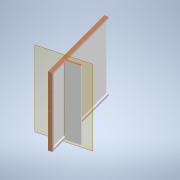
# Autodesk Inventor part: ДИ 00.00.09
Saved by Autodesk Inventor 2021.2 (Build 252289000, 289)
## iProperties
Created: 2021-10-12
Part Number: ДИ 00.00.09
Material: Типовые
Document SubType Name: Modeling
Designer: Surflay
Density: 1 g/cm^3
Appearance: По умолчанию
Author: Surflay
Autodesk Inventor part; units mm, degrees
ref_plane "YZ Plane" through (0, 0, 0) normal (1, 0, 0) x (0, 1, 0)
ref_plane "XZ Plane" through (0, 0, 0) normal (0, 1, 0) x (-1, 0, 0)
ref_plane "XY Plane" through (0, 0, 0) normal (0, 0, 1) x (1, 0, 0)
ref_plane "РабПлоскость1" through (-45, 39.0097, 0) normal (-0.9659258, 0, 0.258819) x (0, -1, 0)
sketch "Эскиз1" plane through (-45, 39.0097, 0) normal (-0.9659258, 0, 0.258819) x (0, -1, 0)
  line L0 (0, 0) -> (78.0194, 0) projected
  line L1 (0.0194, 85.4597) -> (78.0194, 85.4597) projected
  line L2 (78.0194, 68.8953) -> (78.0194, 85.4597) projected
  line L3 (-2.9723, 68.8953) -> (78.0194, 68.8953) projected
  line L4 (-2.9723, 68.8953) -> (-2.9723, 74.9718) projected
  ellipse E0 centre (-19.9806, 77.6951) end of major axis (0.0194, 77.6951) minor radius 5.1764 (-2.9723, 74.9718) -> (0.0194, 77.6951) ccw projected
  line L5 (0.0194, 80.2833) -> (0.0194, 77.6951) projected
  line L6 (0.0194, 80.2833) -> (0.0194, 85.4597) projected
  line L7 (0, 0) -> (78.0194, 0)
  line L8 (78.0194, 0) -> (78.0194, 90.4597)
  line L9 (78.0194, 90.4597) -> (0, 90.4597)
  line L10 (0, 90.4597) -> (0, 0)
  point P0 (39.0097, 11.6469)
  dimension "d1" = 5
  constraints: 8 end point, 2 parallel, 1 horizontal, 1 perpendicular, 1 other
  measures "d1" distance between parallel lines of L1 L9
extrude "Выдавливание1" add sketch "Эскиз1" against normal blind 2 contours L10 L3 L8 L0 | L10 E0 L5 L6 L1 L2 L3 | L10 L9 L8 L1 L6 L5 E0
sketch "Эскиз2" plane through (-43.0681, 39.0097, -0.5176) normal (0.9659258, 0, -0.258819) x (-0.258819, 0, -0.9659258)
  line L0 (0, 0) -> (0, -78.0194) projected
  line L1 (0, -78.0194) -> (-90.4597, -78.0194)
  line L2 (-90.4597, -78.0194) -> (-90.4597, -76.0194)
  line L3 (-90.4597, -76.0194) -> (0, -76.0194)
  line L4 (0, -76.0194) -> (0, -78.0194)
  line L5 (0, 0) -> (-90.4597, 0)
  line L6 (-90.4597, 0) -> (-90.4597, -2)
  line L7 (-90.4597, -2) -> (0, -2)
  line L8 (0, -2) -> (0, 0)
  line L9 (-90.4597, -78.0194) -> (-90.4597, 0) projected
  line L10 (-90.4597, -76.0194) -> (-88.4597, -76.0194)
  line L11 (-88.4597, -76.0194) -> (-88.4597, -2)
  line L12 (-88.4597, -2) -> (-90.4597, -2)
  line L13 (-90.4597, -2) -> (-90.4597, -76.0194)
  line L14 (-66.4597, -76.0194) -> (-68.4597, -76.0194)
  line L15 (-68.4597, -76.0194) -> (-68.4597, -2)
  line L16 (-68.4597, -2) -> (-66.4597, -2)
  line L17 (-66.4597, -2) -> (-66.4597, -76.0194)
  point P0 (-11.6469, -39.0097)
  point P1 (-90.4597, -1)
  point P2 (-90.4597, -77.0194)
  point P3 (-89.4597, -2)
  point P4 (-90.4597, -76.0194)
  point P5 (0, -76.0194)
  point P6 (-66.4597, -2)
  point P7 (0, -2)
  point P8 (-90.4597, -2)
  point P9 (-88.4597, -76.0194)
  point P10 (-88.4597, -2)
  dimension "d4" = 2
  dimension "d5" = 2
  dimension "d6" = 2
  dimension "d7" = 2
  dimension "d8" = 20
  constraints: 32 end point, 8 parallel, 5 point on line, 4 horizontal, 4 perpendicular, 3 midpoint
  measures "d4" distance of L1.end L2.end
  measures "d5" distance of L6.end L5.end
  measures "d6" distance of L12.end L11.end
  measures "d7" distance of L15.end L16.end
  measures "d8" distance between parallel lines of L11 L15
extrude "Выдавливание2" add sketch "Эскиз2" along normal blind 2 contours L0 L7 L6 L5 | L0 L1 L2 L3 | L17 L3 L15 L7 | L7 L11 L3 L9
ref_plane "РабПлоскость2" through (-23.4176, 37.0097, 65.0917) normal (0.258819, 0, 0.9659258) x (0, -1, 0)
sketch "Эскиз3" plane through (-23.4176, 37.0097, 65.0917) normal (0.258819, 0, 0.9659258) x (0, -1, 0)
  line L0 (-2, 0) -> (76.0194, 0) projected
  point P0 (37.0097, 39.4667)
sketch "Эскиз4" plane through (-23.4176, 37.0097, 65.0917) normal (0.258819, 0, 0.9659258) x (0, -1, 0)
  line L0 (76.0194, 0) -> (-2, 0)
  line L1 (-2, 0) -> (-2, 15)
  line L2 (-2, 15) -> (76.0194, 15)
  line L3 (76.0194, 15) -> (76.0194, 0)
  point P0 (37.0097, 39.4667)
  dimension "d12" = 15
  constraints: 8 end point, 2 parallel, 1 horizontal, 1 perpendicular
  measures "d12" distance of L0.end L1.end
extrude "Выдавливание3" add sketch "Эскиз4" along normal blind 2
